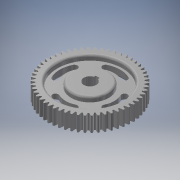
# Autodesk Inventor part: Engranaje recto2
Saved by Autodesk Inventor 2018 (Build 220112000, 112)
## iProperties
Created: 2017-08-08
Part Number: Engranaje recto2
Material: Steel
Document SubType Name: Modeling
Designer: Alumno
Categories: <?xml version="1.0" encoding="UTF-16"?> <MemberInstance><Categories><FamilyTemplate><FamilyTemplateParameter ValueType="xs:double" Id="1" ObjectReferenceKey="da_z" ObjectType="kUserParameterObject"/><FamilyTemplateParameter ValueType="xs:double" Id="2" ObjectReferenceKey="da_b" ObjectType="kUserParameterObject"/><FamilyTemplateParameter ValueType="xs:double" Id="3" ObjectReferenceKey="da_beta" ObjectType="kUserParameterObject"/><FamilyTemplateParameter ValueType="xs:double" Id="4" ObjectReferenceKey="da_da" ObjectType="kUserParameterObject"/><FamilyTemplateParameter ValueType="xs:double" Id="5" ObjectReferenceKey="da_aw" ObjectType="kUserParameterObject"/><FamilyTemplateParameter ValueType="xs:string" Id="6" ObjectReferenceKey="EAIAABAAAACIAQAAAAAAAIAAAAAAAAAA" ObjectType="83910656" SubObjectId="SurfaceGeometry"/></FamilyTemplate><ParamToTemplateMap><ParamToTemplate CategoryParameter="//CategoryParameter[@InternalName='046C89C9-8512-4d59-83FE-43B91F4F132A']" TemplateParameter="1"/><ParamToTemplate CategoryParameter="//CategoryParameter[@InternalName='2552DF32-E462-4b46-AEBF-C6C7768E72AC']" TemplateParameter="2"/><ParamToTemplate CategoryParameter="//CategoryParameter[@InternalName='C9EE641D-15FC-4fae-A226-E94C4372FDD7']" TemplateParameter="3"/><ParamToTemplate><ParamToTemplate CategoryParameter="//CategoryParameter[@InternalName='00B6519A-459B-49c7-AD84-2E56D39A5744']" ConstantValue="0.000000"/></ParamToTemplate><ParamToTemplate><ParamToTemplate CategoryParameter="//CategoryParameter[@InternalName='04B31F0E-C7A6-4894-AA32-9629BEFACF47']" ConstantValue="1.000000"/></ParamToTemplate><ParamToTemplate><ParamToTemplate CategoryParameter="//CategoryParameter[@InternalName='43CBEC2E-7847-49e7-A936-2F7889FCB2D9']" ConstantValue="0.250000"/></ParamToTemplate><ParamToTemplate><ParamToTemplate CategoryParameter="//CategoryParameter[@InternalName='B1EFC894-105D-4ebd-86BF-FA20ED196853']" ConstantValue="0.350000"/></ParamToTemplate><ParamToTemplate><ParamToTemplate CategoryParameter="//CategoryParameter[@InternalName='51175063-3D10-4879-93E8-6246FE8B403D']" ConstantValue="2060000000.000000"/></ParamToTemplate><ParamToTemplate><ParamToTemplate CategoryParameter="//CategoryParameter[@InternalName='A3A52E27-4454-46a9-B0BD-C932399B70AF']" ConstantValue="0.300000"/></ParamToTemplate><ParamToTemplate><ParamToTemplate CategoryParameter="//CategoryParameter[@InternalName='91B76062-C214-41d9-B1B9-14D2AB99603D']" ConstantValue="0.300000"/></ParamToTemplate><ParamToTemplate><ParamToTemplate CategoryParameter="//CategoryParameter[@InternalName='374E806E-8B8A-4dda-A9AA-1039D6500AD2']" ConstantValue="3.333333"/></ParamToTemplate><ParamToTemplate><ParamToTemplate CategoryParameter="//CategoryParameter[@InternalName='2D373A89-B862-43d6-8D0B-0CBF12AB9F6C']" ConstantValue="0.349066"/></ParamToTemplate><ParamToTemplate CategoryParameter="//CategoryParameter[@InternalName='37777632-D6A2-4fac-9D53-DB8ACD95C989']" TemplateParameter="4"/><ParamToTemplate CategoryParameter="//CategoryParameter[@InternalName='FD1017F1-B727-4f7e-9707-0F86F1FF9423']" TemplateParameter="5"/><ParamToTemplate><ParamToTemplate CategoryParameter="//CategoryParameter[@InternalName='9E1B4470-B2D3-4ff1-B813-535BB4CDF51A']" ConstantValue="3520000.000000"/></ParamToTemplate><ParamToTemplate><ParamToTemplate CategoryParameter="//CategoryParameter[@InternalName='F8452263-BFF6-458c-9FB1-07C4B99E95CD']" ConstantValue="11400000.000000"/></ParamToTemplate><ParamToTemplate><ParamToTemplate CategoryParameter="//CategoryParameter[@InternalName='3E3BB259-FD49-497f-8171-6EBC954A3479']" ConstantValue="2.000000"/></ParamToTemplate><ParamToTemplate CategoryParameter="//CategoryParameter[@InternalName='27C3BAF2-7550-4e4b-AE2C-0DB134B7D9B7']" TemplateParameter="6"/></ParamToTemplateMap><Category DisplayName="Gear" InternalName="DC85795E-93AB-48d5-8EEE-5A27447B64BD" Mnemonic="Gear"><CategoryParameter DisplayName="z" InternalName="046C89C9-8512-4d59-83FE-43B91F4F132A" Mnemonic="z"/><CategoryParameter DisplayName="b" InternalName="2552DF32-E462-4b46-AEBF-C6C7768E72AC" Mnemonic="b"/><CategoryParameter DisplayName="||b|" InternalName="C9EE641D-15FC-4fae-A226-E94C4372FDD7" Mnemonic="beta"/><CategoryParameter DisplayName="x" InternalName="00B6519A-459B-49c7-AD84-2E56D39A5744" Mnemonic="x"/><CategoryParameter DisplayName="a*" InternalName="04B31F0E-C7A6-4894-AA32-9629BEFACF47" Mnemonic="a"/><CategoryParameter DisplayName="c*" InternalName="43CBEC2E-7847-49e7-A936-2F7889FCB2D9" Mnemonic="c"/><CategoryParameter DisplayName="r|.f|*" InternalName="B1EFC894-105D-4ebd-86BF-FA20ED196853" Mnemonic="rf"/><CategoryParameter DisplayName="E" InternalName="51175063-3D10-4879-93E8-6246FE8B403D" Mnemonic="E"/><CategoryParameter DisplayName="||m|" InternalName="A3A52E27-4454-46a9-B0BD-C932399B70AF" Mnemonic="mi"/><Category DisplayName="SpurGear" InternalName="26C5A22E-A91E-4dfd-A3B3-23CCAFAE1764" Mnemonic="SpurGear"><CategoryParameter DisplayName="m" InternalName="91B76062-C214-41d9-B1B9-14D2AB99603D" Mnemonic="m"/><CategoryParameter DisplayName="P" InternalName="374E806E-8B8A-4dda-A9AA-1039D6500AD2" Mnemonic="PP"/><CategoryParameter DisplayName="||a|" InternalName="2D373A89-B862-43d6-8D0B-0CBF12AB9F6C" Mnemonic="alpha"/><CategoryParameter DisplayName="d|.a|" InternalName="37777632-D6A2-4fac-9D53-DB8ACD95C989" Mnemonic="da"/><CategoryParameter DisplayName="a|.w|" InternalName="FD1017F1-B727-4f7e-9707-0F86F1FF9423" Mnemonic="aw"/><CategoryParameter DisplayName="||s||.Flim|" InternalName="9E1B4470-B2D3-4ff1-B813-535BB4CDF51A" Mnemonic="sFlim"/><CategoryParameter DisplayName="||s||.Hlim|" InternalName="F8452263-BFF6-458c-9FB1-07C4B99E95CD" Mnemonic="sHlim"/><CategoryParameter DisplayName="tipo" InternalName="3E3BB259-FD49-497f-8171-6EBC954A3479" Mnemonic="type"/><CategoryParameter DisplayName="PitchDiameter" InternalName="27C3BAF2-7550-4e4b-AE2C-0DB134B7D9B7" Mnemonic="IDS_PITCHDIAM"/></Category></Category></Categories></MemberInstance>
Density: 1 g/cm^3
Appearance: Steel
CustomPartVersion: 1
Author: Alumno
Autodesk Inventor part; units mm, degrees
sketch "Sketch1" plane through (0, 0, 0) normal (0, 0, 1) x (1, 0, 0)
  circle A0 centre (0, 0) radius 84
  dimension "d0" = 168
  constraints: 1 centre point
  measures "d0" diameter of A0
extrude "Extrusion1" add sketch "Sketch1" along normal blind 30
ref_plane "Work Plane2" through (0, 0, 15) normal (0, 0, 1) x (1, 0, 0)
sketch "Sketch2" plane through (0, 0, 0) normal (0, 0, -1) x (-1, 0, 0)
  circle A0 centre (0, 0) radius 84 projected
  circle A1 centre (0, 0) radius 81
  dimension "d3" = 162
  constraints: 1 centre point, 1 coincident
  measures "d3" diameter of A1
surface extrude "Diámetro de separación" sketch "Sketch2" against normal through all shown no curves A1
ref_plane "Work Plane8" through (0, 0, 0) normal (0.9983082, 0.0581448, 0) x (0, 0, 1)
ref_plane "Work Plane9" through (0, 0, 0) normal (1, 0, 0) x (0, 1, 0)
spur gear teeth "Engranaje recto" teeth 54 pitch diameter 162 tip diameter 168 root diameter 154.5 face width 30 start plane through (0, 0, 0) normal (0, 0, -1) x (-1, 0, 0)
sketch "Boceto3" plane through (0, 0, 30) normal (0, 0, 1) x (1, 0, 0)
  circle A0 centre (0, 0) radius 12.5
  dimension "d49" = 25
  constraints: 1 centre point, 1 coincident
  measures "d49" diameter of A0
extrude "Extrusión2" cut sketch "Boceto3" against normal up to surface (30 mm away)
sketch "Boceto4" plane through (0, 0, 30) normal (0, 0, 1) x (1, 0, 0)
  circle A0 centre (0, 0) radius 12.5 projected
  arc A1 (-10.9642, 83.2814) -> (-12.3065, 76.2634) centre (24.3275, 72.8941) ccw projected
  arc A2 (-12.3065, 76.2634) -> (-14.5194, 75.8733) centre (0, 0) ccw projected
  arc A3 (-14.5194, 75.8733) -> (-18.1809, 82.0089) centre (-47.7916, 60.1776) ccw projected
  arc A4 (-18.1809, 82.0089) -> (-20.5584, 81.4454) centre (0, 0) ccw projected
  arc A5 (-20.5584, 81.4454) -> (-21.0769, 74.3191) centre (15.7005, 75.2255) ccw projected
  arc A6 (-21.0769, 74.3191) -> (-23.2295, 73.6746) centre (0, 0) ccw projected
  arc A7 (-23.2295, 73.6746) -> (-27.5786, 79.3437) centre (-54.4547, 54.2224) ccw projected
  arc A8 (-27.5786, 79.3437) -> (-29.8747, 78.508) centre (0, 0) ccw projected
  arc A9 (-29.8747, 78.508) -> (-29.5623, 71.3697) centre (6.8612, 76.5396) ccw projected
  arc A10 (-29.5623, 71.3697) -> (-31.6256, 70.4797) centre (0, 0) ccw projected
  arc A11 (-31.6256, 70.4797) -> (-36.6034, 75.6055) centre (-60.3813, 47.534) ccw projected
  arc A12 (-36.6034, 75.6055) -> (-38.7869, 74.5089) centre (0, 0) ccw projected
  arc A13 (-38.7869, 74.5089) -> (-37.6479, 67.4551) centre (-2.0709, 76.8186) ccw projected
  arc A14 (-37.6479, 67.4551) -> (-39.5939, 66.3316) centre (0, 0) ccw projected
  arc A15 (-39.5939, 66.3316) -> (-45.1332, 70.8449) centre (-65.4914, 40.2027) ccw projected
  arc A16 (-45.1332, 70.8449) -> (-47.1746, 69.5022) centre (0, 0) ccw projected
  arc A17 (-47.1746, 69.5022) -> (-45.2244, 62.6284) centre (-10.975, 76.0587) ccw projected
  arc A18 (-45.2244, 62.6284) -> (-47.0268, 61.2865) centre (0, 0) ccw projected
  arc A19 (-47.0268, 61.2865) -> (-53.0526, 65.1262) centre (-69.7158, 32.3278) ccw projected
  arc A20 (-53.0526, 65.1262) -> (-54.9243, 63.5556) centre (0, 0) ccw projected
  arc A21 (-54.9243, 63.5556) -> (-52.1893, 56.9547) centre (-19.7307, 74.2703) ccw projected
  arc A22 (-52.1893, 56.9547) -> (-53.8238, 55.4127) centre (0, 0) ccw projected
  arc A23 (-53.8238, 55.4127) -> (-60.2546, 58.5268) centre (-72.9974, 24.0157) ccw projected
  arc A24 (-60.2546, 58.5268) -> (-61.9313, 56.7496) centre (0, 0) ccw projected
  arc A25 (-61.9313, 56.7496) -> (-58.4485, 50.5108) centre (-28.2195, 71.4775) ccw projected
  arc A26 (-58.4485, 50.5108) -> (-59.8929, 48.7894) centre (0, 0) ccw projected
  arc A27 (-59.8929, 48.7894) -> (-66.6417, 51.136) centre (-75.2919, 15.3788) ccw projected
  arc A28 (-66.6417, 51.136) -> (-68.1008, 49.1761) centre (0, 0) ccw projected
  arc A29 (-68.1008, 49.1761) -> (-63.9172, 43.3838) centre (-36.3267, 67.7182) ccw projected
  arc A30 (-63.9172, 43.3838) -> (-65.152, 41.5064) centre (0, 0) ccw projected
  arc A31 (-65.152, 41.5064) -> (-72.1276, 43.0536) centre (-76.5682, 6.534) ccw projected
  arc A32 (-72.1276, 43.0536) -> (-73.3493, 40.9375) centre (0, 0) ccw projected
  arc A33 (-73.3493, 40.9375) -> (-68.5216, 35.6701) centre (-43.9427, 63.043) ccw projected
  arc A34 (-68.5216, 35.6701) -> (-69.5301, 33.6621) centre (0, 0) ccw projected
  arc A35 (-69.5301, 33.6621) -> (-76.6381, 34.389) centre (-76.809, -2.3992) ccw projected
  arc A36 (-76.6381, 34.389) -> (-77.6059, 32.1454) centre (0, 0) ccw projected
  arc A37 (-77.6059, 32.1454) -> (-72.1993, 27.474) centre (-50.9644, 57.5153) ccw projected
  arc A38 (-72.1993, 27.474) -> (-72.9678, 25.3625) centre (0, 0) ccw projected
  arc A39 (-72.9678, 25.3625) -> (-80.1122, 25.2593) centre (-76.0111, -11.3) ccw projected
  arc A40 (-80.1122, 25.2593) -> (-80.813, 22.9186) centre (0, 0) ccw projected
  arc A41 (-80.813, 22.9186) -> (-74.9007, 18.9064) centre (-57.2969, 51.2098) ccw projected
  arc A42 (-74.9007, 18.9064) -> (-75.4189, 16.72) centre (0, 0) ccw projected
  arc A43 (-75.4189, 16.72) -> (-82.503, 15.788) centre (-74.1853, -20.0479) ccw projected
  arc A44 (-82.503, 15.788) -> (-82.9272, 13.3818) centre (0, 0) ccw projected
  arc A45 (-82.9272, 13.3818) -> (-76.5891, 10.0831) centre (-62.8546, 44.2117) ccw projected
  arc A46 (-76.5891, 10.0831) -> (-76.85, 7.8513) centre (0, 0) ccw projected
  arc A47 (-76.85, 7.8513) -> (-83.778, 6.1033) centre (-71.3563, -28.5247) ccw projected
  arc A48 (-83.778, 6.1033) -> (-83.9201, 3.664) centre (0, 0) ccw projected
  arc A49 (-83.9201, 3.664) -> (-77.2418, 1.1235) centre (-67.5623, 36.6158) ccw projected
  arc A50 (-77.2418, 1.1235) -> (-77.2418, -1.1235) centre (0, 0) ccw projected
  arc A51 (-77.2418, -1.1235) -> (-83.9201, -3.664) centre (-67.5623, -36.6158) ccw projected
  arc A52 (-83.9201, -3.664) -> (-83.778, -6.1033) centre (0, 0) ccw projected
  arc A53 (-83.778, -6.1033) -> (-76.85, -7.8513) centre (-71.3563, 28.5247) ccw projected
  arc A54 (-76.85, -7.8513) -> (-76.5891, -10.0831) centre (0, 0) ccw projected
  arc A55 (-76.5891, -10.0831) -> (-82.9272, -13.3818) centre (-62.8546, -44.2117) ccw projected
  arc A56 (-82.9272, -13.3818) -> (-82.503, -15.788) centre (0, 0) ccw projected
  arc A57 (-82.503, -15.788) -> (-75.4189, -16.72) centre (-74.1853, 20.0479) ccw projected
  arc A58 (-75.4189, -16.72) -> (-74.9007, -18.9064) centre (0, 0) ccw projected
  arc A59 (-74.9007, -18.9064) -> (-80.813, -22.9186) centre (-57.2969, -51.2098) ccw projected
  arc A60 (-80.813, -22.9186) -> (-80.1122, -25.2593) centre (0, 0) ccw projected
  arc A61 (-80.1122, -25.2593) -> (-72.9678, -25.3625) centre (-76.0111, 11.3) ccw projected
  arc A62 (-72.9678, -25.3625) -> (-72.1993, -27.474) centre (0, 0) ccw projected
  arc A63 (-72.1993, -27.474) -> (-77.6059, -32.1454) centre (-50.9644, -57.5153) ccw projected
  arc A64 (-77.6059, -32.1454) -> (-76.6381, -34.389) centre (0, 0) ccw projected
  arc A65 (-76.6381, -34.389) -> (-69.5301, -33.6621) centre (-76.809, 2.3992) ccw projected
  arc A66 (-69.5301, -33.6621) -> (-68.5216, -35.6701) centre (0, 0) ccw projected
  arc A67 (-68.5216, -35.6701) -> (-73.3493, -40.9375) centre (-43.9427, -63.043) ccw projected
  arc A68 (-73.3493, -40.9375) -> (-72.1276, -43.0536) centre (0, 0) ccw projected
  arc A69 (-72.1276, -43.0536) -> (-65.152, -41.5064) centre (-76.5682, -6.534) ccw projected
  arc A70 (-65.152, -41.5064) -> (-63.9172, -43.3838) centre (0, 0) ccw projected
  arc A71 (-63.9172, -43.3838) -> (-68.1008, -49.1761) centre (-36.3267, -67.7182) ccw projected
  arc A72 (-68.1008, -49.1761) -> (-66.6417, -51.136) centre (0, 0) ccw projected
  arc A73 (-66.6417, -51.136) -> (-59.8929, -48.7894) centre (-75.2919, -15.3788) ccw projected
  arc A74 (-59.8929, -48.7894) -> (-58.4485, -50.5108) centre (0, 0) ccw projected
  arc A75 (-58.4485, -50.5108) -> (-61.9313, -56.7496) centre (-28.2195, -71.4775) ccw projected
  arc A76 (-61.9313, -56.7496) -> (-60.2546, -58.5268) centre (0, 0) ccw projected
  arc A77 (-60.2546, -58.5268) -> (-53.8238, -55.4127) centre (-72.9974, -24.0157) ccw projected
  arc A78 (-53.8238, -55.4127) -> (-52.1893, -56.9547) centre (0, 0) ccw projected
  arc A79 (-52.1893, -56.9547) -> (-54.9243, -63.5556) centre (-19.7307, -74.2703) ccw projected
  arc A80 (-54.9243, -63.5556) -> (-53.0526, -65.1262) centre (0, 0) ccw projected
  arc A81 (-53.0526, -65.1262) -> (-47.0268, -61.2865) centre (-69.7158, -32.3278) ccw projected
  arc A82 (-47.0268, -61.2865) -> (-45.2244, -62.6284) centre (0, 0) ccw projected
  arc A83 (-45.2244, -62.6284) -> (-47.1746, -69.5022) centre (-10.975, -76.0587) ccw projected
  arc A84 (-47.1746, -69.5022) -> (-45.1332, -70.8449) centre (0, 0) ccw projected
  arc A85 (-45.1332, -70.8449) -> (-39.5939, -66.3316) centre (-65.4914, -40.2027) ccw projected
  arc A86 (-39.5939, -66.3316) -> (-37.6479, -67.4551) centre (0, 0) ccw projected
  arc A87 (-37.6479, -67.4551) -> (-38.7869, -74.5089) centre (-2.0709, -76.8186) ccw projected
  arc A88 (-38.7869, -74.5089) -> (-36.6034, -75.6055) centre (0, 0) ccw projected
  arc A89 (-36.6034, -75.6055) -> (-31.6256, -70.4797) centre (-60.3813, -47.534) ccw projected
  arc A90 (-31.6256, -70.4797) -> (-29.5623, -71.3697) centre (0, 0) ccw projected
  arc A91 (-29.5623, -71.3697) -> (-29.8747, -78.508) centre (6.8612, -76.5396) ccw projected
  arc A92 (-29.8747, -78.508) -> (-27.5786, -79.3437) centre (0, 0) ccw projected
  arc A93 (-27.5786, -79.3437) -> (-23.2295, -73.6746) centre (-54.4547, -54.2224) ccw projected
  arc A94 (-23.2295, -73.6746) -> (-21.0769, -74.3191) centre (0, 0) ccw projected
  arc A95 (-21.0769, -74.3191) -> (-20.5584, -81.4454) centre (15.7005, -75.2255) ccw projected
  arc A96 (-20.5584, -81.4454) -> (-18.1809, -82.0089) centre (0, 0) ccw projected
  arc A97 (-18.1809, -82.0089) -> (-14.5194, -75.8733) centre (-47.7916, -60.1776) ccw projected
  arc A98 (-14.5194, -75.8733) -> (-12.3065, -76.2634) centre (0, 0) ccw projected
  arc A99 (-12.3065, -76.2634) -> (-10.9642, -83.2814) centre (24.3275, -72.8941) ccw projected
  arc A100 (-10.9642, -83.2814) -> (-8.5373, -83.565) centre (0, 0) ccw projected
  arc A101 (-8.5373, -83.565) -> (-5.6128, -77.0458) centre (-40.4823, -65.3189) ccw projected
  arc A102 (-5.6128, -77.0458) -> (-3.3696, -77.1765) centre (0, 0) ccw projected
  arc A103 (-3.3696, -77.1765) -> (-1.2217, -83.9911) centre (32.6255, -69.577) ccw projected
  arc A104 (-1.2217, -83.9911) -> (1.2217, -83.9911) centre (0, 0) ccw projected
  arc A105 (1.2217, -83.9911) -> (3.3696, -77.1765) centre (-32.6255, -69.577) ccw projected
  arc A106 (3.3696, -77.1765) -> (5.6128, -77.0458) centre (0, 0) ccw projected
  arc A107 (5.6128, -77.0458) -> (8.5373, -83.565) centre (40.4823, -65.3189) ccw projected
  arc A108 (8.5373, -83.565) -> (10.9642, -83.2814) centre (0, 0) ccw projected
  arc A109 (10.9642, -83.2814) -> (12.3065, -76.2634) centre (-24.3275, -72.8941) ccw projected
  arc A110 (12.3065, -76.2634) -> (14.5194, -75.8733) centre (0, 0) ccw projected
  arc A111 (14.5194, -75.8733) -> (18.1809, -82.0089) centre (47.7916, -60.1776) ccw projected
  arc A112 (18.1809, -82.0089) -> (20.5584, -81.4454) centre (0, 0) ccw projected
  arc A113 (20.5584, -81.4454) -> (21.0769, -74.3191) centre (-15.7005, -75.2255) ccw projected
  arc A114 (21.0769, -74.3191) -> (23.2295, -73.6746) centre (0, 0) ccw projected
  arc A115 (23.2295, -73.6746) -> (27.5786, -79.3437) centre (54.4547, -54.2224) ccw projected
  arc A116 (27.5786, -79.3437) -> (29.8747, -78.508) centre (0, 0) ccw projected
  arc A117 (29.8747, -78.508) -> (29.5623, -71.3697) centre (-6.8612, -76.5396) ccw projected
  arc A118 (29.5623, -71.3697) -> (31.6256, -70.4797) centre (0, 0) ccw projected
  arc A119 (31.6256, -70.4797) -> (36.6034, -75.6055) centre (60.3813, -47.534) ccw projected
  arc A120 (36.6034, -75.6055) -> (38.7869, -74.5089) centre (0, 0) ccw projected
  arc A121 (38.7869, -74.5089) -> (37.6479, -67.4551) centre (2.0709, -76.8186) ccw projected
  arc A122 (37.6479, -67.4551) -> (39.5939, -66.3316) centre (0, 0) ccw projected
  arc A123 (39.5939, -66.3316) -> (45.1332, -70.8449) centre (65.4914, -40.2027) ccw projected
  arc A124 (45.1332, -70.8449) -> (47.1746, -69.5022) centre (0, 0) ccw projected
  arc A125 (47.1746, -69.5022) -> (45.2244, -62.6284) centre (10.975, -76.0587) ccw projected
  arc A126 (45.2244, -62.6284) -> (47.0268, -61.2865) centre (0, 0) ccw projected
  arc A127 (47.0268, -61.2865) -> (53.0526, -65.1262) centre (69.7158, -32.3278) ccw projected
  arc A128 (53.0526, -65.1262) -> (54.9243, -63.5556) centre (0, 0) ccw projected
  arc A129 (54.9243, -63.5556) -> (52.1893, -56.9547) centre (19.7307, -74.2703) ccw projected
  arc A130 (52.1893, -56.9547) -> (53.8238, -55.4127) centre (0, 0) ccw projected
  arc A131 (53.8238, -55.4127) -> (60.2546, -58.5268) centre (72.9974, -24.0157) ccw projected
  arc A132 (60.2546, -58.5268) -> (61.9313, -56.7496) centre (0, 0) ccw projected
  arc A133 (61.9313, -56.7496) -> (58.4485, -50.5108) centre (28.2195, -71.4775) ccw projected
  arc A134 (58.4485, -50.5108) -> (59.8929, -48.7894) centre (0, 0) ccw projected
  arc A135 (59.8929, -48.7894) -> (66.6417, -51.136) centre (75.2919, -15.3788) ccw projected
  arc A136 (66.6417, -51.136) -> (68.1008, -49.1761) centre (0, 0) ccw projected
  arc A137 (68.1008, -49.1761) -> (63.9172, -43.3838) centre (36.3267, -67.7182) ccw projected
  arc A138 (63.9172, -43.3838) -> (65.152, -41.5064) centre (0, 0) ccw projected
  arc A139 (65.152, -41.5064) -> (72.1276, -43.0536) centre (76.5682, -6.534) ccw projected
  arc A140 (72.1276, -43.0536) -> (73.3493, -40.9375) centre (0, 0) ccw projected
  arc A141 (73.3493, -40.9375) -> (68.5216, -35.6701) centre (43.9427, -63.043) ccw projected
  arc A142 (68.5216, -35.6701) -> (69.5301, -33.6621) centre (0, 0) ccw projected
  arc A143 (69.5301, -33.6621) -> (76.6381, -34.389) centre (76.809, 2.3992) ccw projected
  arc A144 (76.6381, -34.389) -> (77.6059, -32.1454) centre (0, 0) ccw projected
  arc A145 (77.6059, -32.1454) -> (72.1993, -27.474) centre (50.9644, -57.5153) ccw projected
  arc A146 (72.1993, -27.474) -> (72.9678, -25.3625) centre (0, 0) ccw projected
  arc A147 (72.9678, -25.3625) -> (80.1122, -25.2593) centre (76.0111, 11.3) ccw projected
  arc A148 (80.1122, -25.2593) -> (80.813, -22.9186) centre (0, 0) ccw projected
  arc A149 (80.813, -22.9186) -> (74.9007, -18.9064) centre (57.2969, -51.2098) ccw projected
  arc A150 (74.9007, -18.9064) -> (75.4189, -16.72) centre (0, 0) ccw projected
  arc A151 (75.4189, -16.72) -> (82.503, -15.788) centre (74.1853, 20.0479) ccw projected
  arc A152 (82.503, -15.788) -> (82.9272, -13.3818) centre (0, 0) ccw projected
  arc A153 (82.9272, -13.3818) -> (76.5891, -10.0831) centre (62.8546, -44.2117) ccw projected
  arc A154 (76.5891, -10.0831) -> (76.85, -7.8513) centre (0, 0) ccw projected
  arc A155 (76.85, -7.8513) -> (83.778, -6.1033) centre (71.3563, 28.5247) ccw projected
  arc A156 (83.778, -6.1033) -> (83.9201, -3.664) centre (0, 0) ccw projected
  arc A157 (83.9201, -3.664) -> (77.2418, -1.1235) centre (67.5623, -36.6158) ccw projected
  arc A158 (77.2418, -1.1235) -> (77.2418, 1.1235) centre (0, 0) ccw projected
  arc A159 (77.2418, 1.1235) -> (83.9201, 3.664) centre (67.5623, 36.6158) ccw projected
  arc A160 (83.9201, 3.664) -> (83.778, 6.1033) centre (0, 0) ccw projected
  arc A161 (83.778, 6.1033) -> (76.85, 7.8513) centre (71.3563, -28.5247) ccw projected
  arc A162 (76.85, 7.8513) -> (76.5891, 10.0831) centre (0, 0) ccw projected
  arc A163 (76.5891, 10.0831) -> (82.9272, 13.3818) centre (62.8546, 44.2117) ccw projected
  arc A164 (82.9272, 13.3818) -> (82.503, 15.788) centre (0, 0) ccw projected
  arc A165 (82.503, 15.788) -> (75.4189, 16.72) centre (74.1853, -20.0479) ccw projected
  arc A166 (75.4189, 16.72) -> (74.9007, 18.9064) centre (0, 0) ccw projected
  arc A167 (74.9007, 18.9064) -> (80.813, 22.9186) centre (57.2969, 51.2098) ccw projected
  arc A168 (80.813, 22.9186) -> (80.1122, 25.2593) centre (0, 0) ccw projected
  arc A169 (80.1122, 25.2593) -> (72.9678, 25.3625) centre (76.0111, -11.3) ccw projected
  arc A170 (72.9678, 25.3625) -> (72.1993, 27.474) centre (0, 0) ccw projected
  arc A171 (72.1993, 27.474) -> (77.6059, 32.1454) centre (50.9644, 57.5153) ccw projected
  arc A172 (77.6059, 32.1454) -> (76.6381, 34.389) centre (0, 0) ccw projected
  arc A173 (76.6381, 34.389) -> (69.5301, 33.6621) centre (76.809, -2.3992) ccw projected
  arc A174 (69.5301, 33.6621) -> (68.5216, 35.6701) centre (0, 0) ccw projected
  arc A175 (68.5216, 35.6701) -> (73.3493, 40.9375) centre (43.9427, 63.043) ccw projected
  arc A176 (73.3493, 40.9375) -> (72.1276, 43.0536) centre (0, 0) ccw projected
  arc A177 (72.1276, 43.0536) -> (65.152, 41.5064) centre (76.5682, 6.534) ccw projected
  arc A178 (65.152, 41.5064) -> (63.9172, 43.3838) centre (0, 0) ccw projected
  arc A179 (63.9172, 43.3838) -> (68.1008, 49.1761) centre (36.3267, 67.7182) ccw projected
  arc A180 (68.1008, 49.1761) -> (66.6417, 51.136) centre (0, 0) ccw projected
  arc A181 (66.6417, 51.136) -> (59.8929, 48.7894) centre (75.2919, 15.3788) ccw projected
  arc A182 (59.8929, 48.7894) -> (58.4485, 50.5108) centre (0, 0) ccw projected
  arc A183 (58.4485, 50.5108) -> (61.9313, 56.7496) centre (28.2195, 71.4775) ccw projected
  arc A184 (61.9313, 56.7496) -> (60.2546, 58.5268) centre (0, 0) ccw projected
  arc A185 (60.2546, 58.5268) -> (53.8238, 55.4127) centre (72.9974, 24.0157) ccw projected
  arc A186 (53.8238, 55.4127) -> (52.1893, 56.9547) centre (0, 0) ccw projected
  arc A187 (52.1893, 56.9547) -> (54.9243, 63.5556) centre (19.7307, 74.2703) ccw projected
  arc A188 (54.9243, 63.5556) -> (53.0526, 65.1262) centre (0, 0) ccw projected
  arc A189 (53.0526, 65.1262) -> (47.0268, 61.2865) centre (69.7158, 32.3278) ccw projected
  arc A190 (47.0268, 61.2865) -> (45.2244, 62.6284) centre (0, 0) ccw projected
  arc A191 (45.2244, 62.6284) -> (47.1746, 69.5022) centre (10.975, 76.0587) ccw projected
  arc A192 (47.1746, 69.5022) -> (45.1332, 70.8449) centre (0, 0) ccw projected
  arc A193 (45.1332, 70.8449) -> (39.5939, 66.3316) centre (65.4914, 40.2027) ccw projected
  arc A194 (39.5939, 66.3316) -> (37.6479, 67.4551) centre (0, 0) ccw projected
  arc A195 (37.6479, 67.4551) -> (38.7869, 74.5089) centre (2.0709, 76.8186) ccw projected
  arc A196 (38.7869, 74.5089) -> (36.6034, 75.6055) centre (0, 0) ccw projected
  arc A197 (36.6034, 75.6055) -> (31.6256, 70.4797) centre (60.3813, 47.534) ccw projected
  arc A198 (31.6256, 70.4797) -> (29.5623, 71.3697) centre (0, 0) ccw projected
  arc A199 (29.5623, 71.3697) -> (29.8747, 78.508) centre (-6.8612, 76.5396) ccw projected
  arc A200 (29.8747, 78.508) -> (27.5786, 79.3437) centre (0, 0) ccw projected
  arc A201 (27.5786, 79.3437) -> (23.2295, 73.6746) centre (54.4547, 54.2224) ccw projected
  arc A202 (23.2295, 73.6746) -> (21.0769, 74.3191) centre (0, 0) ccw projected
  arc A203 (21.0769, 74.3191) -> (20.5584, 81.4454) centre (-15.7005, 75.2255) ccw projected
  arc A204 (20.5584, 81.4454) -> (18.1809, 82.0089) centre (0, 0) ccw projected
  arc A205 (18.1809, 82.0089) -> (14.5194, 75.8733) centre (47.7916, 60.1776) ccw projected
  arc A206 (14.5194, 75.8733) -> (12.3065, 76.2634) centre (0, 0) ccw projected
  arc A207 (12.3065, 76.2634) -> (10.9642, 83.2814) centre (-24.3275, 72.8941) ccw projected
  arc A208 (10.9642, 83.2814) -> (8.5373, 83.565) centre (0, 0) ccw projected
  arc A209 (8.5373, 83.565) -> (5.6128, 77.0458) centre (40.4823, 65.3189) ccw projected
  arc A210 (5.6128, 77.0458) -> (3.3696, 77.1765) centre (0, 0) ccw projected
  arc A211 (3.3696, 77.1765) -> (1.2217, 83.9911) centre (-32.6255, 69.577) ccw projected
  arc A212 (1.2217, 83.9911) -> (-1.2217, 83.9911) centre (0, 0) ccw projected
  arc A213 (-1.2217, 83.9911) -> (-3.3696, 77.1765) centre (32.6255, 69.577) ccw projected
  arc A214 (-3.3696, 77.1765) -> (-5.6128, 77.0458) centre (0, 0) ccw projected
  arc A215 (-5.6128, 77.0458) -> (-8.5373, 83.565) centre (-40.4823, 65.3189) ccw projected
  arc A216 (-8.5373, 83.565) -> (-10.9642, 83.2814) centre (0, 0) ccw projected
  line L0 (0, 0) -> (0, 12.5)
  line L1 (4, 9.5) -> (-4, 9.5)
  line L2 (-4, 9.5) -> (-4, 15.5)
  line L3 (-4, 15.5) -> (4, 15.5)
  line L4 (4, 15.5) -> (4, 9.5)
  line L5 (4, 9.5) -> (-4, 15.5) construction
  line L6 (-4, 9.5) -> (4, 15.5) construction
  dimension "d52" = 8
  dimension "d53" = 6
  constraints: 14 end point, 2 midpoint, 2 parallel, 1 horizontal, 1 perpendicular, 1 vertical, 1 vertical alignment, 1 other
  measures "d52" distance of L2.end L3.end
  measures "d53" distance of L1.end L2.end
extrude "Extrusión3" cut sketch "Boceto4" against normal up to surface (30 mm away) contours L4 L1 L0 A0 | A0 L2 L3 L4 | A0 L0 L1 L2
sketch "Sketch5" plane through (0, 0, 0) normal (0, 0, -1) x (-1, 0, 0)
  line L0 (4, 15.5) -> (4, 11.8427) projected
  arc A0 (-4, 11.8427) -> (4, 11.8427) centre (0, 0) ccw projected
  line L1 (-4, 11.8427) -> (-4, 15.5) projected
  line L2 (-4, 15.5) -> (4, 15.5) projected
  arc A1 (12.3065, 76.2634) -> (10.9642, 83.2814) centre (-24.3275, 72.8941) ccw projected
  arc A2 (10.9642, 83.2814) -> (8.5373, 83.565) centre (0, 0) ccw projected
  arc A3 (8.5373, 83.565) -> (5.6128, 77.0458) centre (40.4823, 65.3189) ccw projected
  arc A4 (5.6128, 77.0458) -> (3.3696, 77.1765) centre (0, 0) ccw projected
  arc A5 (3.3696, 77.1765) -> (1.2217, 83.9911) centre (-32.6255, 69.577) ccw projected
  arc A6 (1.2217, 83.9911) -> (-1.2217, 83.9911) centre (0, 0) ccw projected
  arc A7 (-1.2217, 83.9911) -> (-3.3696, 77.1765) centre (32.6255, 69.577) ccw projected
  arc A8 (-3.3696, 77.1765) -> (-5.6128, 77.0458) centre (0, 0) ccw projected
  arc A9 (-5.6128, 77.0458) -> (-8.5373, 83.565) centre (-40.4823, 65.3189) ccw projected
  arc A10 (-8.5373, 83.565) -> (-10.9642, 83.2814) centre (0, 0) ccw projected
  arc A11 (-10.9642, 83.2814) -> (-12.3065, 76.2634) centre (24.3275, 72.8941) ccw projected
  arc A12 (-12.3065, 76.2634) -> (-14.5194, 75.8733) centre (0, 0) ccw projected
  arc A13 (-14.5194, 75.8733) -> (-18.1809, 82.0089) centre (-47.7916, 60.1776) ccw projected
  arc A14 (-18.1809, 82.0089) -> (-20.5584, 81.4454) centre (0, 0) ccw projected
  arc A15 (-20.5584, 81.4454) -> (-21.0769, 74.3191) centre (15.7005, 75.2255) ccw projected
  arc A16 (-21.0769, 74.3191) -> (-23.2295, 73.6746) centre (0, 0) ccw projected
  arc A17 (-23.2295, 73.6746) -> (-27.5786, 79.3437) centre (-54.4547, 54.2224) ccw projected
  arc A18 (-27.5786, 79.3437) -> (-29.8747, 78.508) centre (0, 0) ccw projected
  arc A19 (-29.8747, 78.508) -> (-29.5623, 71.3697) centre (6.8612, 76.5396) ccw projected
  arc A20 (-29.5623, 71.3697) -> (-31.6256, 70.4797) centre (0, 0) ccw projected
  arc A21 (-31.6256, 70.4797) -> (-36.6034, 75.6055) centre (-60.3813, 47.534) ccw projected
  arc A22 (-36.6034, 75.6055) -> (-38.7869, 74.5089) centre (0, 0) ccw projected
  arc A23 (-38.7869, 74.5089) -> (-37.6479, 67.4551) centre (-2.0709, 76.8186) ccw projected
  arc A24 (-37.6479, 67.4551) -> (-39.5939, 66.3316) centre (0, 0) ccw projected
  arc A25 (-39.5939, 66.3316) -> (-45.1332, 70.8449) centre (-65.4914, 40.2027) ccw projected
  arc A26 (-45.1332, 70.8449) -> (-47.1746, 69.5022) centre (0, 0) ccw projected
  arc A27 (-47.1746, 69.5022) -> (-45.2244, 62.6284) centre (-10.975, 76.0587) ccw projected
  arc A28 (-45.2244, 62.6284) -> (-47.0268, 61.2865) centre (0, 0) ccw projected
  arc A29 (-47.0268, 61.2865) -> (-53.0526, 65.1262) centre (-69.7158, 32.3278) ccw projected
  arc A30 (-53.0526, 65.1262) -> (-54.9243, 63.5556) centre (0, 0) ccw projected
  arc A31 (-54.9243, 63.5556) -> (-52.1893, 56.9547) centre (-19.7307, 74.2703) ccw projected
  arc A32 (-52.1893, 56.9547) -> (-53.8238, 55.4127) centre (0, 0) ccw projected
  arc A33 (-53.8238, 55.4127) -> (-60.2546, 58.5268) centre (-72.9974, 24.0157) ccw projected
  arc A34 (-60.2546, 58.5268) -> (-61.9313, 56.7496) centre (0, 0) ccw projected
  arc A35 (-61.9313, 56.7496) -> (-58.4485, 50.5108) centre (-28.2195, 71.4775) ccw projected
  arc A36 (-58.4485, 50.5108) -> (-59.8929, 48.7894) centre (0, 0) ccw projected
  arc A37 (-59.8929, 48.7894) -> (-66.6417, 51.136) centre (-75.2919, 15.3788) ccw projected
  arc A38 (-66.6417, 51.136) -> (-68.1008, 49.1761) centre (0, 0) ccw projected
  arc A39 (-68.1008, 49.1761) -> (-63.9172, 43.3838) centre (-36.3267, 67.7182) ccw projected
  arc A40 (-63.9172, 43.3838) -> (-65.152, 41.5064) centre (0, 0) ccw projected
  arc A41 (-65.152, 41.5064) -> (-72.1276, 43.0536) centre (-76.5682, 6.534) ccw projected
  arc A42 (-72.1276, 43.0536) -> (-73.3493, 40.9375) centre (0, 0) ccw projected
  arc A43 (-73.3493, 40.9375) -> (-68.5216, 35.6701) centre (-43.9427, 63.043) ccw projected
  arc A44 (-68.5216, 35.6701) -> (-69.5301, 33.6621) centre (0, 0) ccw projected
  arc A45 (-69.5301, 33.6621) -> (-76.6381, 34.389) centre (-76.809, -2.3992) ccw projected
  arc A46 (-76.6381, 34.389) -> (-77.6059, 32.1454) centre (0, 0) ccw projected
  arc A47 (-77.6059, 32.1454) -> (-72.1993, 27.474) centre (-50.9644, 57.5153) ccw projected
  arc A48 (-72.1993, 27.474) -> (-72.9678, 25.3625) centre (0, 0) ccw projected
  arc A49 (-72.9678, 25.3625) -> (-80.1122, 25.2593) centre (-76.0111, -11.3) ccw projected
  arc A50 (-80.1122, 25.2593) -> (-80.813, 22.9186) centre (0, 0) ccw projected
  arc A51 (-80.813, 22.9186) -> (-74.9007, 18.9064) centre (-57.2969, 51.2098) ccw projected
  arc A52 (-74.9007, 18.9064) -> (-75.4189, 16.72) centre (0, 0) ccw projected
  arc A53 (-75.4189, 16.72) -> (-82.503, 15.788) centre (-74.1853, -20.0479) ccw projected
  arc A54 (-82.503, 15.788) -> (-82.9272, 13.3818) centre (0, 0) ccw projected
  arc A55 (-82.9272, 13.3818) -> (-76.5891, 10.0831) centre (-62.8546, 44.2117) ccw projected
  arc A56 (-76.5891, 10.0831) -> (-76.85, 7.8513) centre (0, 0) ccw projected
  arc A57 (-76.85, 7.8513) -> (-83.778, 6.1033) centre (-71.3563, -28.5247) ccw projected
  arc A58 (-83.778, 6.1033) -> (-83.9201, 3.664) centre (0, 0) ccw projected
  arc A59 (-83.9201, 3.664) -> (-77.2418, 1.1235) centre (-67.5623, 36.6158) ccw projected
  arc A60 (-77.2418, 1.1235) -> (-77.2418, -1.1235) centre (0, 0) ccw projected
  arc A61 (-77.2418, -1.1235) -> (-83.9201, -3.664) centre (-67.5623, -36.6158) ccw projected
  arc A62 (-83.9201, -3.664) -> (-83.778, -6.1033) centre (0, 0) ccw projected
  arc A63 (-83.778, -6.1033) -> (-76.85, -7.8513) centre (-71.3563, 28.5247) ccw projected
  arc A64 (-76.85, -7.8513) -> (-76.5891, -10.0831) centre (0, 0) ccw projected
  arc A65 (-76.5891, -10.0831) -> (-82.9272, -13.3818) centre (-62.8546, -44.2117) ccw projected
  arc A66 (-82.9272, -13.3818) -> (-82.503, -15.788) centre (0, 0) ccw projected
  arc A67 (-82.503, -15.788) -> (-75.4189, -16.72) centre (-74.1853, 20.0479) ccw projected
  arc A68 (-75.4189, -16.72) -> (-74.9007, -18.9064) centre (0, 0) ccw projected
  arc A69 (-74.9007, -18.9064) -> (-80.813, -22.9186) centre (-57.2969, -51.2098) ccw projected
  arc A70 (-80.813, -22.9186) -> (-80.1122, -25.2593) centre (0, 0) ccw projected
  arc A71 (-80.1122, -25.2593) -> (-72.9678, -25.3625) centre (-76.0111, 11.3) ccw projected
  arc A72 (-72.9678, -25.3625) -> (-72.1993, -27.474) centre (0, 0) ccw projected
  arc A73 (-72.1993, -27.474) -> (-77.6059, -32.1454) centre (-50.9644, -57.5153) ccw projected
  arc A74 (-77.6059, -32.1454) -> (-76.6381, -34.389) centre (0, 0) ccw projected
  arc A75 (-76.6381, -34.389) -> (-69.5301, -33.6621) centre (-76.809, 2.3992) ccw projected
  arc A76 (-69.5301, -33.6621) -> (-68.5216, -35.6701) centre (0, 0) ccw projected
  arc A77 (-68.5216, -35.6701) -> (-73.3493, -40.9375) centre (-43.9427, -63.043) ccw projected
  arc A78 (-73.3493, -40.9375) -> (-72.1276, -43.0536) centre (0, 0) ccw projected
  arc A79 (-72.1276, -43.0536) -> (-65.152, -41.5064) centre (-76.5682, -6.534) ccw projected
  arc A80 (-65.152, -41.5064) -> (-63.9172, -43.3838) centre (0, 0) ccw projected
  arc A81 (-63.9172, -43.3838) -> (-68.1008, -49.1761) centre (-36.3267, -67.7182) ccw projected
  arc A82 (-68.1008, -49.1761) -> (-66.6417, -51.136) centre (0, 0) ccw projected
  arc A83 (-66.6417, -51.136) -> (-59.8929, -48.7894) centre (-75.2919, -15.3788) ccw projected
  arc A84 (-59.8929, -48.7894) -> (-58.4485, -50.5108) centre (0, 0) ccw projected
  arc A85 (-58.4485, -50.5108) -> (-61.9313, -56.7496) centre (-28.2195, -71.4775) ccw projected
  arc A86 (-61.9313, -56.7496) -> (-60.2546, -58.5268) centre (0, 0) ccw projected
  arc A87 (-60.2546, -58.5268) -> (-53.8238, -55.4127) centre (-72.9974, -24.0157) ccw projected
  arc A88 (-53.8238, -55.4127) -> (-52.1893, -56.9547) centre (0, 0) ccw projected
  arc A89 (-52.1893, -56.9547) -> (-54.9243, -63.5556) centre (-19.7307, -74.2703) ccw projected
  arc A90 (-54.9243, -63.5556) -> (-53.0526, -65.1262) centre (0, 0) ccw projected
  arc A91 (-53.0526, -65.1262) -> (-47.0268, -61.2865) centre (-69.7158, -32.3278) ccw projected
  arc A92 (-47.0268, -61.2865) -> (-45.2244, -62.6284) centre (0, 0) ccw projected
  arc A93 (-45.2244, -62.6284) -> (-47.1746, -69.5022) centre (-10.975, -76.0587) ccw projected
  arc A94 (-47.1746, -69.5022) -> (-45.1332, -70.8449) centre (0, 0) ccw projected
  arc A95 (-45.1332, -70.8449) -> (-39.5939, -66.3316) centre (-65.4914, -40.2027) ccw projected
  arc A96 (-39.5939, -66.3316) -> (-37.6479, -67.4551) centre (0, 0) ccw projected
  arc A97 (-37.6479, -67.4551) -> (-38.7869, -74.5089) centre (-2.0709, -76.8186) ccw projected
  arc A98 (-38.7869, -74.5089) -> (-36.6034, -75.6055) centre (0, 0) ccw projected
  arc A99 (-36.6034, -75.6055) -> (-31.6256, -70.4797) centre (-60.3813, -47.534) ccw projected
  arc A100 (-31.6256, -70.4797) -> (-29.5623, -71.3697) centre (0, 0) ccw projected
  arc A101 (-29.5623, -71.3697) -> (-29.8747, -78.508) centre (6.8612, -76.5396) ccw projected
  arc A102 (-29.8747, -78.508) -> (-27.5786, -79.3437) centre (0, 0) ccw projected
  arc A103 (-27.5786, -79.3437) -> (-23.2295, -73.6746) centre (-54.4547, -54.2224) ccw projected
  arc A104 (-23.2295, -73.6746) -> (-21.0769, -74.3191) centre (0, 0) ccw projected
  arc A105 (-21.0769, -74.3191) -> (-20.5584, -81.4454) centre (15.7005, -75.2255) ccw projected
  arc A106 (-20.5584, -81.4454) -> (-18.1809, -82.0089) centre (0, 0) ccw projected
  arc A107 (-18.1809, -82.0089) -> (-14.5194, -75.8733) centre (-47.7916, -60.1776) ccw projected
  arc A108 (-14.5194, -75.8733) -> (-12.3065, -76.2634) centre (0, 0) ccw projected
  arc A109 (-12.3065, -76.2634) -> (-10.9642, -83.2814) centre (24.3275, -72.8941) ccw projected
  arc A110 (-10.9642, -83.2814) -> (-8.5373, -83.565) centre (0, 0) ccw projected
  arc A111 (-8.5373, -83.565) -> (-5.6128, -77.0458) centre (-40.4823, -65.3189) ccw projected
  arc A112 (-5.6128, -77.0458) -> (-3.3696, -77.1765) centre (0, 0) ccw projected
  arc A113 (-3.3696, -77.1765) -> (-1.2217, -83.9911) centre (32.6255, -69.577) ccw projected
  arc A114 (-1.2217, -83.9911) -> (1.2217, -83.9911) centre (0, 0) ccw projected
  arc A115 (1.2217, -83.9911) -> (3.3696, -77.1765) centre (-32.6255, -69.577) ccw projected
  arc A116 (3.3696, -77.1765) -> (5.6128, -77.0458) centre (0, 0) ccw projected
  arc A117 (5.6128, -77.0458) -> (8.5373, -83.565) centre (40.4823, -65.3189) ccw projected
  arc A118 (8.5373, -83.565) -> (10.9642, -83.2814) centre (0, 0) ccw projected
  arc A119 (10.9642, -83.2814) -> (12.3065, -76.2634) centre (-24.3275, -72.8941) ccw projected
  arc A120 (12.3065, -76.2634) -> (14.5194, -75.8733) centre (0, 0) ccw projected
  arc A121 (14.5194, -75.8733) -> (18.1809, -82.0089) centre (47.7916, -60.1776) ccw projected
  arc A122 (18.1809, -82.0089) -> (20.5584, -81.4454) centre (0, 0) ccw projected
  arc A123 (20.5584, -81.4454) -> (21.0769, -74.3191) centre (-15.7005, -75.2255) ccw projected
  arc A124 (21.0769, -74.3191) -> (23.2295, -73.6746) centre (0, 0) ccw projected
  arc A125 (23.2295, -73.6746) -> (27.5786, -79.3437) centre (54.4547, -54.2224) ccw projected
  arc A126 (27.5786, -79.3437) -> (29.8747, -78.508) centre (0, 0) ccw projected
  arc A127 (29.8747, -78.508) -> (29.5623, -71.3697) centre (-6.8612, -76.5396) ccw projected
  arc A128 (29.5623, -71.3697) -> (31.6256, -70.4797) centre (0, 0) ccw projected
  arc A129 (31.6256, -70.4797) -> (36.6034, -75.6055) centre (60.3813, -47.534) ccw projected
  arc A130 (36.6034, -75.6055) -> (38.7869, -74.5089) centre (0, 0) ccw projected
  arc A131 (38.7869, -74.5089) -> (37.6479, -67.4551) centre (2.0709, -76.8186) ccw projected
  arc A132 (37.6479, -67.4551) -> (39.5939, -66.3316) centre (0, 0) ccw projected
  arc A133 (39.5939, -66.3316) -> (45.1332, -70.8449) centre (65.4914, -40.2027) ccw projected
  arc A134 (45.1332, -70.8449) -> (47.1746, -69.5022) centre (0, 0) ccw projected
  arc A135 (47.1746, -69.5022) -> (45.2244, -62.6284) centre (10.975, -76.0587) ccw projected
  arc A136 (45.2244, -62.6284) -> (47.0268, -61.2865) centre (0, 0) ccw projected
  arc A137 (47.0268, -61.2865) -> (53.0526, -65.1262) centre (69.7158, -32.3278) ccw projected
  arc A138 (53.0526, -65.1262) -> (54.9243, -63.5556) centre (0, 0) ccw projected
  arc A139 (54.9243, -63.5556) -> (52.1893, -56.9547) centre (19.7307, -74.2703) ccw projected
  arc A140 (52.1893, -56.9547) -> (53.8238, -55.4127) centre (0, 0) ccw projected
  arc A141 (53.8238, -55.4127) -> (60.2546, -58.5268) centre (72.9974, -24.0157) ccw projected
  arc A142 (60.2546, -58.5268) -> (61.9313, -56.7496) centre (0, 0) ccw projected
  arc A143 (61.9313, -56.7496) -> (58.4485, -50.5108) centre (28.2195, -71.4775) ccw projected
  arc A144 (58.4485, -50.5108) -> (59.8929, -48.7894) centre (0, 0) ccw projected
  arc A145 (59.8929, -48.7894) -> (66.6417, -51.136) centre (75.2919, -15.3788) ccw projected
  arc A146 (66.6417, -51.136) -> (68.1008, -49.1761) centre (0, 0) ccw projected
  arc A147 (68.1008, -49.1761) -> (63.9172, -43.3838) centre (36.3267, -67.7182) ccw projected
  arc A148 (63.9172, -43.3838) -> (65.152, -41.5064) centre (0, 0) ccw projected
  arc A149 (65.152, -41.5064) -> (72.1276, -43.0536) centre (76.5682, -6.534) ccw projected
  arc A150 (72.1276, -43.0536) -> (73.3493, -40.9375) centre (0, 0) ccw projected
  arc A151 (73.3493, -40.9375) -> (68.5216, -35.6701) centre (43.9427, -63.043) ccw projected
  arc A152 (68.5216, -35.6701) -> (69.5301, -33.6621) centre (0, 0) ccw projected
  arc A153 (69.5301, -33.6621) -> (76.6381, -34.389) centre (76.809, 2.3992) ccw projected
  arc A154 (76.6381, -34.389) -> (77.6059, -32.1454) centre (0, 0) ccw projected
  arc A155 (77.6059, -32.1454) -> (72.1993, -27.474) centre (50.9644, -57.5153) ccw projected
  arc A156 (72.1993, -27.474) -> (72.9678, -25.3625) centre (0, 0) ccw projected
  arc A157 (72.9678, -25.3625) -> (80.1122, -25.2593) centre (76.0111, 11.3) ccw projected
  arc A158 (80.1122, -25.2593) -> (80.813, -22.9186) centre (0, 0) ccw projected
  arc A159 (80.813, -22.9186) -> (74.9007, -18.9064) centre (57.2969, -51.2098) ccw projected
  arc A160 (74.9007, -18.9064) -> (75.4189, -16.72) centre (0, 0) ccw projected
  arc A161 (75.4189, -16.72) -> (82.503, -15.788) centre (74.1853, 20.0479) ccw projected
  arc A162 (82.503, -15.788) -> (82.9272, -13.3818) centre (0, 0) ccw projected
  arc A163 (82.9272, -13.3818) -> (76.5891, -10.0831) centre (62.8546, -44.2117) ccw projected
  arc A164 (76.5891, -10.0831) -> (76.85, -7.8513) centre (0, 0) ccw projected
  arc A165 (76.85, -7.8513) -> (83.778, -6.1033) centre (71.3563, 28.5247) ccw projected
  arc A166 (83.778, -6.1033) -> (83.9201, -3.664) centre (0, 0) ccw projected
  arc A167 (83.9201, -3.664) -> (77.2418, -1.1235) centre (67.5623, -36.6158) ccw projected
  arc A168 (77.2418, -1.1235) -> (77.2418, 1.1235) centre (0, 0) ccw projected
  arc A169 (77.2418, 1.1235) -> (83.9201, 3.664) centre (67.5623, 36.6158) ccw projected
  arc A170 (83.9201, 3.664) -> (83.778, 6.1033) centre (0, 0) ccw projected
  arc A171 (83.778, 6.1033) -> (76.85, 7.8513) centre (71.3563, -28.5247) ccw projected
  arc A172 (76.85, 7.8513) -> (76.5891, 10.0831) centre (0, 0) ccw projected
  arc A173 (76.5891, 10.0831) -> (82.9272, 13.3818) centre (62.8546, 44.2117) ccw projected
  arc A174 (82.9272, 13.3818) -> (82.503, 15.788) centre (0, 0) ccw projected
  arc A175 (82.503, 15.788) -> (75.4189, 16.72) centre (74.1853, -20.0479) ccw projected
  arc A176 (75.4189, 16.72) -> (74.9007, 18.9064) centre (0, 0) ccw projected
  arc A177 (74.9007, 18.9064) -> (80.813, 22.9186) centre (57.2969, 51.2098) ccw projected
  arc A178 (80.813, 22.9186) -> (80.1122, 25.2593) centre (0, 0) ccw projected
  arc A179 (80.1122, 25.2593) -> (72.9678, 25.3625) centre (76.0111, -11.3) ccw projected
  arc A180 (72.9678, 25.3625) -> (72.1993, 27.474) centre (0, 0) ccw projected
  arc A181 (72.1993, 27.474) -> (77.6059, 32.1454) centre (50.9644, 57.5153) ccw projected
  arc A182 (77.6059, 32.1454) -> (76.6381, 34.389) centre (0, 0) ccw projected
  arc A183 (76.6381, 34.389) -> (69.5301, 33.6621) centre (76.809, -2.3992) ccw projected
  arc A184 (69.5301, 33.6621) -> (68.5216, 35.6701) centre (0, 0) ccw projected
  arc A185 (68.5216, 35.6701) -> (73.3493, 40.9375) centre (43.9427, 63.043) ccw projected
  arc A186 (73.3493, 40.9375) -> (72.1276, 43.0536) centre (0, 0) ccw projected
  arc A187 (72.1276, 43.0536) -> (65.152, 41.5064) centre (76.5682, 6.534) ccw projected
  arc A188 (65.152, 41.5064) -> (63.9172, 43.3838) centre (0, 0) ccw projected
  arc A189 (63.9172, 43.3838) -> (68.1008, 49.1761) centre (36.3267, 67.7182) ccw projected
  arc A190 (68.1008, 49.1761) -> (66.6417, 51.136) centre (0, 0) ccw projected
  arc A191 (66.6417, 51.136) -> (59.8929, 48.7894) centre (75.2919, 15.3788) ccw projected
  arc A192 (59.8929, 48.7894) -> (58.4485, 50.5108) centre (0, 0) ccw projected
  arc A193 (58.4485, 50.5108) -> (61.9313, 56.7496) centre (28.2195, 71.4775) ccw projected
  arc A194 (61.9313, 56.7496) -> (60.2546, 58.5268) centre (0, 0) ccw projected
  arc A195 (60.2546, 58.5268) -> (53.8238, 55.4127) centre (72.9974, 24.0157) ccw projected
  arc A196 (53.8238, 55.4127) -> (52.1893, 56.9547) centre (0, 0) ccw projected
  arc A197 (52.1893, 56.9547) -> (54.9243, 63.5556) centre (19.7307, 74.2703) ccw projected
  arc A198 (54.9243, 63.5556) -> (53.0526, 65.1262) centre (0, 0) ccw projected
  arc A199 (53.0526, 65.1262) -> (47.0268, 61.2865) centre (69.7158, 32.3278) ccw projected
  arc A200 (47.0268, 61.2865) -> (45.2244, 62.6284) centre (0, 0) ccw projected
  arc A201 (45.2244, 62.6284) -> (47.1746, 69.5022) centre (10.975, 76.0587) ccw projected
  arc A202 (47.1746, 69.5022) -> (45.1332, 70.8449) centre (0, 0) ccw projected
  arc A203 (45.1332, 70.8449) -> (39.5939, 66.3316) centre (65.4914, 40.2027) ccw projected
  arc A204 (39.5939, 66.3316) -> (37.6479, 67.4551) centre (0, 0) ccw projected
  arc A205 (37.6479, 67.4551) -> (38.7869, 74.5089) centre (2.0709, 76.8186) ccw projected
  arc A206 (38.7869, 74.5089) -> (36.6034, 75.6055) centre (0, 0) ccw projected
  arc A207 (36.6034, 75.6055) -> (31.6256, 70.4797) centre (60.3813, 47.534) ccw projected
  arc A208 (31.6256, 70.4797) -> (29.5623, 71.3697) centre (0, 0) ccw projected
  arc A209 (29.5623, 71.3697) -> (29.8747, 78.508) centre (-6.8612, 76.5396) ccw projected
  arc A210 (29.8747, 78.508) -> (27.5786, 79.3437) centre (0, 0) ccw projected
  arc A211 (27.5786, 79.3437) -> (23.2295, 73.6746) centre (54.4547, 54.2224) ccw projected
  arc A212 (23.2295, 73.6746) -> (21.0769, 74.3191) centre (0, 0) ccw projected
  arc A213 (21.0769, 74.3191) -> (20.5584, 81.4454) centre (-15.7005, 75.2255) ccw projected
  arc A214 (20.5584, 81.4454) -> (18.1809, 82.0089) centre (0, 0) ccw projected
  arc A215 (18.1809, 82.0089) -> (14.5194, 75.8733) centre (47.7916, 60.1776) ccw projected
  arc A216 (14.5194, 75.8733) -> (12.3065, 76.2634) centre (0, 0) ccw projected
  circle A217 centre (0, 0) radius 65
  circle A218 centre (0, 0) radius 37.5
  dimension "d56" = 130
  dimension "d57" = 75
  constraints: 2 centre point, 2 coincident
  measures "d56" diameter of A217
  measures "d57" diameter of A218
extrude "Extrusion4" cut sketch "Sketch5" against normal blind 10 contours A217
fillet "Fillet2" radius 4 2 edges at (37.5, 0, 0) (65, 0, 0)
ref_plane "Work Plane11" through (0, 0, 15) normal (0, 0, -1) x (-1, 0, 0)
mirror "Mirror1" about plane through (0, 0, 15) normal (0, 0, -1) of "Extrusion4"
mirror "Mirror2" about plane through (0, 0, 15) normal (0, 0, -1) of "Fillet2"
sketch "Sketch6" plane through (0, 0, 20) normal (0, 0, 1) x (1, 0, 0)
  circle A0 centre (0, 0) radius 70
  arc A1 (16.3559, 44.623) -> (21.6806, 55.377) centre (19.0182, 50) ccw
  arc A2 (16.3559, 44.623) -> (-16.3559, 44.623) centre (0, 11.5902) ccw
  arc A3 (-21.6806, 55.377) -> (-16.3559, 44.623) centre (-19.0182, 50) ccw
  arc A4 (21.6806, 55.377) -> (-21.6806, 55.377) centre (0, 11.5902) ccw
  arc A5 (-44.623, 16.3559) -> (-55.377, 21.6806) centre (-50, 19.0182) ccw
  arc A6 (-44.623, 16.3559) -> (-44.623, -16.3559) centre (-11.5902, 0) ccw
  arc A7 (-55.377, -21.6806) -> (-44.623, -16.3559) centre (-50, -19.0182) ccw
  arc A8 (-55.377, 21.6806) -> (-55.377, -21.6806) centre (-11.5902, 0) ccw
  arc A9 (-16.3559, -44.623) -> (-21.6806, -55.377) centre (-19.0182, -50) ccw
  arc A10 (-16.3559, -44.623) -> (16.3559, -44.623) centre (0, -11.5902) ccw
  arc A11 (21.6806, -55.377) -> (16.3559, -44.623) centre (19.0182, -50) ccw
  arc A12 (-21.6806, -55.377) -> (21.6806, -55.377) centre (0, -11.5902) ccw
  arc A13 (44.623, -16.3559) -> (55.377, -21.6806) centre (50, -19.0182) ccw
  arc A14 (44.623, -16.3559) -> (44.623, 16.3559) centre (11.5902, 0) ccw
  arc A15 (55.377, 21.6806) -> (44.623, 16.3559) centre (50, 19.0182) ccw
  arc A16 (55.377, -21.6806) -> (55.377, 21.6806) centre (11.5902, 0) ccw
  circle A17 centre (0, 0) radius 31
  constraints: 32 point on circle, 18 centre point
extrude "Extrusion5" cut sketch "Sketch6" against normal up to surface (10 mm away) contours A2 A3 A4 A1 | A6 A7 A8 A5 | A10 A11 A12 A9 | A14 A15 A16 A13
equation "\"d0\" = da_da"
equation "\"d1\" = da_b"
equation "\"d3\" = da_dw"
equation "\"d16\" = da_aw"
equation "\"d43\" = da_aw"
equation "\"d46\" = da_aw"
equation "\"da_da\" = 168"
equation "\"da_b\" = 30"
equation "\"da_dw\" = 162"
equation "\"da_aw\" = 108"
body "Solid1"
body "Srf1"
